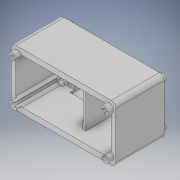
# Autodesk Inventor part: servo midden
Saved by Autodesk Inventor 2019 (Build 230136000, 136)
## iProperties
Created: 2021-01-14
Part Number: servo midden
Material: Glass
Document SubType Name: Modeling
Designer: CS
Density: 2.18 g/cm^3
Appearance: Default
Author: CS
Autodesk Inventor part; units mm, degrees
ref_plane "YZ Plane" through (0, 0, 0) normal (1, 0, 0) x (0, 1, 0)
ref_plane "XZ Plane" through (0, 0, 0) normal (0, 1, 0) x (-1, 0, 0)
ref_plane "XY Plane" through (0, 0, 0) normal (0, 0, 1) x (1, 0, 0)
sketch "Sketch1" plane through (0, 0, 0) normal (0, 0, 1) x (1, 0, 0)
  line L0 (-11.375, -6.1) -> (11.375, -6.1)
  line L1 (11.375, -6.1) -> (11.375, 6.1)
  line L2 (11.375, 6.1) -> (-11.375, 6.1)
  line L3 (-11.375, 6.1) -> (-11.375, -6.1)
  line L4 (-11.375, -6.1) -> (11.375, 6.1) construction
  line L5 (11.375, -6.1) -> (-11.375, 6.1) construction
  line L6 (10, -4.5) -> (-10, -4.5) construction
  line L7 (-10, -4.5) -> (-10, 4.5) construction
  line L8 (-10, 4.5) -> (10, 4.5) construction
  line L9 (10, 4.5) -> (10, -4.5) construction
  line L10 (10, -4.5) -> (-10, 4.5) construction
  line L11 (-10, -4.5) -> (10, 4.5) construction
  circle A0 centre (-10, 4.5) radius 0.5
  circle A1 centre (-10, -4.5) radius 0.5
  circle A2 centre (10, -4.5) radius 0.5
  circle A3 centre (10, 4.5) radius 0.5
  circle A4 centre (-10, 4.5) radius 0.875
  circle A5 centre (10, 4.5) radius 0.875
  circle A6 centre (10, -4.5) radius 0.875
  circle A7 centre (-10, -4.5) radius 0.875
  point P0 (0, 0)
  dimension "d0" = 22.75
  dimension "d1" = 12.2
  dimension "d2" = 9
  dimension "d3" = 20
  dimension "d4" = 1
  dimension "d6" = 1.75
  constraints: 24 end point, 8 centre point, 6 equal radius, 4 coincident, 4 midpoint, 4 parallel, 2 horizontal, 2 perpendicular
  measures "d0" distance of L1.end L2.end
  measures "d1" distance of L0.end L1.end
  measures "d2" distance of L8.end L6.start
  measures "d3" distance of L7.end L8.end
  measures "d4" diameter of A0
  measures "d6" diameter of A4
extrude "Extrusion1" add sketch "Sketch1" along normal blind 10.5 contours L3 L2 L1 L0 | A4 | A5 | A6 | A7
fillet "Fillet1" radius 1 4 edges at (11.375, 6.1, 5.25) (-11.375, 6.1, 5.25) (11.375, -6.1, 5.25) (-11.375, -6.1, 5.25)
extrude "Extrusion2" add sketch "Sketch1" against normal blind 1 contours A4 | A5 | A6 | A7
extrude "Extrusion3" add sketch "Sketch1" along normal blind 1 from surface at 10.5 contours A4 | A5 | A6 | A7
sketch "Sketch2" plane through (0, 0, 10.5) normal (0, 0, 1) x (1, 0, 0)
  line L0 (8.975, -4.9) -> (-8.975, -4.9)
  line L1 (-10.375, -3.5) -> (-10.375, 3.5)
  line L2 (-8.975, 4.9) -> (8.975, 4.9)
  line L3 (10.375, 3.5) -> (10.375, -3.5)
  line L4 (10.375, -4.9) -> (-10.375, 4.9) construction
  line L5 (-10.375, -4.9) -> (10.375, 4.9) construction
  line L6 (10.375, 6.1) -> (-10.375, 6.1) projected
  line L7 (11.375, -5.1) -> (11.375, 5.1) projected
  line L8 (8.975, 4.9) -> (10.375, 3.5)
  line L9 (-10.375, 3.5) -> (-8.975, 4.9)
  line L10 (-8.975, -4.9) -> (-10.375, -3.5)
  arc A0 (-10.375, 6.1) -> (-11.375, 5.1) centre (-10.375, 5.1) ccw projected
  line L11 (-11.375, 5.1) -> (-11.375, -5.1) projected
  arc A1 (-11.375, -5.1) -> (-10.375, -6.1) centre (-10.375, -5.1) ccw projected
  line L12 (-10.375, -6.1) -> (10.375, -6.1) projected
  arc A2 (10.375, -6.1) -> (11.375, -5.1) centre (10.375, -5.1) ccw projected
  arc A3 (11.375, 5.1) -> (10.375, 6.1) centre (10.375, 5.1) ccw projected
  line L13 (8.975, -4.9) -> (10.375, -3.5)
  point P0 (0, 0)
  dimension "d15" = 1.2
  dimension "d16" = 1
  dimension "d17" = 1.4
  dimension "d18" = 1.4
  dimension "d19" = 1.4
  dimension "d20" = 1.4
  dimension "d21" = 1.4
  dimension "d22" = 1.4
  dimension "d32" = 1.4
  dimension "d33" = 1.4
  constraints: 20 end point, 8 point on line, 2 midpoint, 2 parallel, 1 horizontal, 1 perpendicular
  measures "d15" distance between parallel lines of L6 L2
  measures "d16" distance between parallel lines of L7 L3
  measures "d17" distance of L2.end L5.end
  measures "d18" distance of L3.start L5.end
  measures "d19" distance of L1.end L4.end
  measures "d20" distance of L2.start L4.end
  measures "d21" distance of L0.end L5.start
  measures "d22" distance of L1.start L5.start
  measures "d32" distance of L0.start L4.start
  measures "d33" distance of L3.end L4.start
extrude "Extrusion6" cut sketch "Sketch2" along normal blind 2 and the other way blind 9 contours L0 L10 L1 L9 L2 L8 L3 L13
fillet "Fillet2" radius 0.01 8 edges at (-9.8529, 4.0221, 6.5) (-9.5221, 4.3529, 6.5) (-9.8529, -4.0221, 6.5) (-9.5221, -4.3529, 6.5) (9.5221, 4.3529, 6.5) (9.8529, 4.0221, 6.5) (9.5221, -4.3529, 6.5) (9.8529, -4.0221, 6.5)
sketch "Sketch3" plane through (0, 0, 1.5) normal (0, 0, 1) x (1, 0, 0)
  line L0 (-8.975, 4.9) -> (8.975, 4.9) construction
  line L1 (-10.375, -3.5) -> (-10.375, 3.5) construction
  line L2 (8.975, -4.9) -> (-8.975, -4.9) construction
  line L3 (10.375, 3.5) -> (10.375, -3.5) construction
  line L4 (2.375, 4.9) -> (1.625, 4.9)
  line L5 (1.625, 4.9) -> (1.625, -4.9)
  line L6 (1.625, -4.9) -> (2.375, -4.9)
  line L7 (2.375, -4.9) -> (2.375, 4.9)
  line L8 (1.625, 3.5) -> (1.875, 3.5)
  line L9 (1.875, 3.5) -> (1.875, -3.5)
  line L10 (1.875, -3.5) -> (1.625, -3.5)
  line L11 (1.625, -3.5) -> (1.625, 3.5)
  line L12 (1.625, 1) -> (0.6, 1)
  arc A0 (0.6, 1) -> (0.6, -1) centre (0.6, 0) ccw
  line L13 (0.6, -1) -> (1.625, -1)
  line L14 (-6.625, 5.35) -> (-3.125, 5.35)
  line L15 (-3.125, 5.35) -> (-3.125, 3.35)
  line L16 (-3.125, 3.35) -> (-6.625, 3.35)
  line L17 (-6.625, 3.35) -> (-6.625, 5.35)
  line L18 (-6.625, -5.35) -> (-3.125, -5.35)
  line L19 (-3.125, -5.35) -> (-3.125, -3.35)
  line L20 (-3.125, -3.35) -> (-6.625, -3.35)
  line L21 (-6.625, -3.35) -> (-6.625, -5.35)
  line L22 (10.375, 6.1) -> (-10.375, 6.1) projected
  line L23 (-10.375, -6.1) -> (10.375, -6.1) projected
  line L24 (-11.375, 5.1) -> (-11.375, -5.1) projected
  point P0 (0, 0)
  point P1 (1.875, 0)
  point P2 (1.625, 0)
  dimension "d34" = 0.75
  dimension "d35" = 12
  dimension "d36" = 7
  dimension "d37" = 0.25
  dimension "d38" = 2
  dimension "d39" = 1.025
  dimension "d46" = 0.75
  dimension "d47" = 0.75
  dimension "d48" = 2
  dimension "d49" = 3.5
  dimension "d50" = 4.75
  constraints: 36 end point, 8 parallel, 6 perpendicular, 5 point on line, 4 horizontal, 2 equal length, 2 horizontal alignment, 2 midpoint, 2 point on circle, 2 tangent, 1 centre point, 1 collinear
  measures "d34" distance between parallel lines of L7 L5
  measures "d35" distance between parallel lines of L1 L5
  measures "d36" distance of L8.end L9.end
  measures "d37" distance between parallel lines of L11 L9
  measures "d38" distance between parallel lines of L13 L12
  measures "d39" distance from line of L11 A0.centre
  measures "d46" distance between parallel lines of L22 L14
  measures "d47" distance between parallel lines of L23 L18
  measures "d48" distance of L14.end L15.end
  measures "d49" distance of L15.end L16.end
  measures "d50" distance between parallel lines of L24 L17
extrude "Extrusion7" add sketch "Sketch3" along normal blind 6.5 contours L7 L6 L5 L10 L9 L8 L4
sketch "Sketch4" plane through (0, 0, 1.5) normal (0, 0, 1) x (1, 0, 0)
  line L0 (2.375, 4.9) -> (2.375, -4.9) projected
  line L1 (8.975, -4.9) -> (2.375, -4.9) projected
  line L2 (9.4958, -4.3792) -> (8.975, -4.9) projected
  line L3 (10.375, 3.5) -> (10.375, -3.5) projected
  line L4 (9.8792, 3.9958) -> (10.375, 3.5) projected
  line L5 (2.375, 4.9) -> (8.975, 4.9) projected
  circle A0 centre (6.625, 0) radius 2
  line L6 (11.375, -5.1) -> (11.375, 5.1) projected
  arc A1 (9.5126, -4.3885) -> (9.4958, -4.3792) centre (9.5028, -4.3863) ccw projected
  arc A2 (9.8885, -4.0126) -> (9.5126, -4.3885) centre (10, -4.5) ccw projected
  arc A3 (9.8792, -3.9958) -> (9.8885, -4.0126) centre (9.8863, -4.0028) ccw projected
  line L7 (10.375, -3.5) -> (9.8792, -3.9958) projected
  arc A4 (9.8885, 4.0126) -> (9.8792, 3.9958) centre (9.8863, 4.0028) ccw projected
  arc A5 (9.5126, 4.3885) -> (9.8885, 4.0126) centre (10, 4.5) ccw projected
  arc A6 (9.4958, 4.3792) -> (9.5126, 4.3885) centre (9.5028, 4.3863) ccw projected
  line L8 (8.975, 4.9) -> (9.4958, 4.3792) projected
  point P0 (0, 0)
  dimension "d75" = 4
  dimension "d77" = 4.75
  constraints: 1 centre point, 1 horizontal alignment
  measures "d75" diameter of A0
  measures "d77" distance from line of L6 A0.centre
extrude "Extrusion9" add sketch "Sketch3" along normal blind 1 contours L8 L9 L10 L5 | L5 L13 A0 L12
extrude "Extrusion10" cut sketch "Sketch3" against normal blind 2 and the other way blind 1 contours L14 L15 L16 L17 | L21 L20 L19 L18
sketch "Sketch6" plane through (0, 0, 0) normal (0, 0, -1) x (-1, 0, 0)
  circle A0 centre (5.375, 0) radius 2.5 construction
  circle A1 centre (-0.6, 0) radius 0.625 projected
  circle A2 centre (5.375, 0) radius 0.625
  circle A3 centre (5.375, 0) radius 1.25
  point P0 (0, 0)
  dimension "d59" = 1.25
  dimension "d60" = 2.5
  constraints: 2 centre point, 2 coincident
  measures "d59" diameter of A2
  measures "d60" diameter of A3
extrude "Extrusion15" cut sketch "Sketch6" against normal up to surface (1.5 mm away) contours A2
sketch "Sketch7" plane through (0, 0, 0) normal (0, 0, -1) x (-1, 0, 0)
  circle A0 centre (5.375, 0) radius 1.25 projected
  circle A1 centre (5.375, 0) radius 0.625 projected
  point P0 (0, 0)
extrude "Extrusion16" add sketch "Sketch7" along normal blind 2
sketch "Sketch8" plane through (0, 0, 0) normal (0, 0, -1) x (-1, 0, 0)
  circle A0 centre (-0.6, 0) radius 0.625 projected
  circle A1 centre (-0.6, 0) radius 0.575
  circle A2 centre (-0.6, 0) radius 1
  point P0 (0, 0)
  dimension "d69" = 1.15
  dimension "d70" = 2
  constraints: 2 centre point, 2 coincident
  measures "d69" diameter of A1
  measures "d70" diameter of A2
extrude "Extrusion17" cut sketch "Sketch8" against normal blind 0.5 contours A1
extrude "Extrusion18" add sketch "Sketch8" along normal blind 0.25 contours A0 | A2
extrude "Extrusion19" cut sketch "Sketch4" against normal blind 0.75
extrude "Extrusion20" cut sketch "Sketch4" against normal through all contours A0
sketch "Sketch9" plane through (0, 0, 1.5) normal (0, 0, 1) x (1, 0, 0)
  circle A0 centre (-5.375, 0) radius 0.625 projected
  line L0 (-3.125, 4.9) -> (-3.125, 3.35) projected
  line L1 (-3.125, 3.35) -> (-6.625, 3.35) projected
  line L2 (-6.625, 3.35) -> (-6.625, 4.9) projected
  line L3 (-8.975, 4.9) -> (-6.625, 4.9) projected
  line L4 (-9.4958, 4.3792) -> (-8.975, 4.9) projected
  line L5 (-10.375, -3.5) -> (-10.375, 3.5) projected
  line L6 (-9.8792, -3.9958) -> (-10.375, -3.5) projected
  line L7 (1.625, -4.9) -> (-3.125, -4.9) projected
  line L8 (-6.625, -4.9) -> (-6.625, -3.35) projected
  line L9 (-6.625, -3.35) -> (-3.125, -3.35) projected
  line L10 (-3.125, -3.35) -> (-3.125, -4.9) projected
  line L11 (-6.625, -4.9) -> (-8.975, -4.9) projected
  line L12 (1.625, -4.9) -> (1.625, -1) projected
  line L13 (1.625, -1) -> (0.6, -1) projected
  arc A1 (0.6, 1) -> (0.6, -1) centre (0.6, 0) ccw projected
  line L14 (0.6, 1) -> (1.625, 1) projected
  line L15 (1.625, 1) -> (1.625, 4.9) projected
  line L16 (-3.125, 4.9) -> (1.625, 4.9) projected
  circle A2 centre (-5.375, 0) radius 2.5
  circle A3 centre (-5.375, 0) radius 0.625 projected
  circle A4 centre (-5.375, 0) radius 3
  line L17 (-8.625, 3.85) -> (-0.625, 3.85) construction
  line L18 (-0.625, 3.85) -> (-0.625, -3.85) construction
  line L19 (-0.625, -3.85) -> (-8.625, -3.85) construction
  line L20 (-8.625, -3.85) -> (-8.625, 3.85) construction
  line L21 (-11.375, 5.1) -> (-11.375, -5.1) construction
  circle A5 centre (-8.625, 3.85) radius 0.875
  circle A6 centre (-8.625, -3.85) radius 0.875
  circle A7 centre (-0.625, 3.85) radius 0.875
  circle A8 centre (-0.625, -3.85) radius 0.875
  arc A9 (-9.5126, 4.3885) -> (-9.4958, 4.3792) centre (-9.5028, 4.3863) ccw projected
  arc A10 (-9.8885, 4.0126) -> (-9.5126, 4.3885) centre (-10, 4.5) ccw projected
  arc A11 (-9.8792, 3.9958) -> (-9.8885, 4.0126) centre (-9.8863, 4.0028) ccw projected
  line L22 (-10.375, 3.5) -> (-9.8792, 3.9958) projected
  arc A12 (-9.8885, -4.0126) -> (-9.8792, -3.9958) centre (-9.8863, -4.0028) ccw projected
  arc A13 (-9.5126, -4.3885) -> (-9.8885, -4.0126) centre (-10, -4.5) ccw projected
  arc A14 (-9.4958, -4.3792) -> (-9.5126, -4.3885) centre (-9.5028, -4.3863) ccw projected
  line L23 (-8.975, -4.9) -> (-9.4958, -4.3792) projected
  line L24 (10.375, 6.1) -> (-10.375, 6.1) projected
  circle A15 centre (-8.625, 3.85) radius 0.575
  circle A16 centre (-8.625, -3.85) radius 0.575
  circle A17 centre (-0.625, 3.85) radius 0.575
  point P0 (0, 0)
  point P1 (-8.625, 0)
  dimension "d82" = 5
  dimension "d83" = 6
  dimension "d86" = 8
  dimension "d89" = 2.75
  dimension "d90" = 1.75
  dimension "d95" = 2.25
  dimension "d96" = 1.15
  constraints: 9 centre point, 9 coincident, 8 end point, 5 equal radius, 2 parallel, 1 horizontal, 1 horizontal alignment, 1 midpoint, 1 perpendicular
  measures "d82" diameter of A2
  measures "d83" diameter of A4
  measures "d86" distance of L17.start L17.end
  measures "d89" distance between parallel lines of L21 L20
  measures "d90" diameter of A5
  measures "d95" distance between parallel lines of L24 L17
  measures "d96" diameter of A15
extrude "Extrusion21" add sketch "Sketch9" along normal blind 1 contours A4
extrude "Extrusion22" add sketch "Sketch9" along normal blind 1 contours A5 | A6 | A7 | A8
sketch "Sketch10" plane through (0, 0, 0) normal (0, 0, -1) x (-1, 0, 0)
  circle A0 centre (-0.6, 0) radius 0.575 projected
  circle A1 centre (-0.6, 0) radius 1 projected
  circle A2 centre (-0.6, 0) radius 5.375
  point P0 (0, 0)
  dimension "d97" = 10.75
  constraints: 1 centre point, 1 coincident
  measures "d97" diameter of A2
extrude "Extrusion23" cut sketch "Sketch10" along normal up to surface (2 mm away) contours A2
equation "\"d18\" = d17"
equation "\"d19\" = d17"
equation "\"d20\" = d19"
equation "\"d21\" = d17"
equation "\"d22\" = d21"
equation "\"d32\" = d17"
equation "\"d33\" = d32"
equation "\"d47\" = d46"
body "Solid1"
